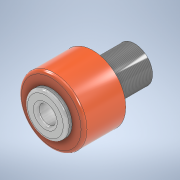
# Autodesk Inventor part: Banana Hembra
Saved by Autodesk Inventor 2020 (Build 240168000, 168)
## iProperties
Created: 2022-05-20
Part Number: Banana Hembra
Material: Generic
Document SubType Name: Modeling
Designer: juanc
Density: 1 g/cm^3
Appearance: Default
Author: juanc
Autodesk Inventor part; units mm, degrees
ref_plane "YZ Plane" through (0, 0, 0) normal (1, 0, 0) x (0, 1, 0)
ref_plane "XZ Plane" through (0, 0, 0) normal (0, 1, 0) x (-1, 0, 0)
ref_plane "XY Plane" through (0, 0, 0) normal (0, 0, 1) x (1, 0, 0)
sketch "Sketch1" plane through (0, 0, 0) normal (0, 0, 1) x (1, 0, 0)
  circle A0 centre (0, 0) radius 139.7
  dimension "d0" = 279.4
  constraints: 1 centre point, 1 coincident
  measures "d0" diameter of A0
extrude "Extrusion1" add sketch "Sketch1" along normal blind 177.8
sketch "Sketch2" plane through (0, 0, 177.8) normal (0, 0, 1) x (1, 0, 0)
  circle A0 centre (0, 0) radius 88.9
  dimension "d3" = 177.8
  constraints: 1 centre point, 1 coincident
  measures "d3" diameter of A0
extrude "Extrusion2" add sketch "Sketch2" along normal blind 25.4
fillet "Fillet1" radius 12.7 1 edges at (-139.7, 0, 177.8)
fillet "Fillet2" radius 12.7 1 edges at (-88.9, 0, 203.2)
sketch "Sketch3" plane through (0, 0, 203.2) normal (0, 0, 1) x (1, 0, 0)
  circle A0 centre (0, 0) radius 127 projected
  circle A1 centre (0, 0) radius 38.1
  dimension "d8" = 76.2
  constraints: 1 centre point, 1 coincident
  measures "d8" diameter of A1
hole "Hole1" at (0, 0, 203.2) direction (0, 0, -1) diameter 76.2 end through all
fillet "Fillet3" radius 12.7 1 edges at (0, 38.1, 203.2)
sketch "Sketch4" plane through (0, 0, 0) normal (0, 0, -1) x (-1, 0, 0)
  circle A0 centre (0, 0) radius 38.1
  circle A1 centre (0, 0) radius 76.2
  dimension "d17" = 152.4
  constraints: 2 centre point, 2 coincident
  measures "d17" diameter of A1
extrude "Extrusion3" add sketch "Sketch4" along normal blind 177.8
thread "Thread1" size "30-318 UNM" class "2A" standard "ANSI Unified Screw Threads" full length
thread "Thread2" size "M155x6" class "6g" standard "ANSI Metric M Profile" full length
body "Solid1"
